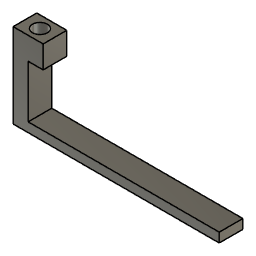
_Hook v2.cb20e67a-e10a-452d-a86b-8f95d06309be (Autodesk Fusion 360 design; units mm, degrees)
part number: 2025-05-20-10-46-20-879
part number: 2025-05-20-11-01-20-780
Autodesk Fusion 360 part; units mm, degrees
sketch "Sketch1" plane through (0, 0, 0) normal (0, 0, 1) x (1, 0, 0)
  line L0 (0, 0) -> (55, 0)
  line L1 (55, 0) -> (55, 6.3)
  line L2 (55, 6.3) -> (0, 6.3)
  line L3 (0, 6.3) -> (0, 0)
  dimension "d1" = 55
  dimension "d2" = 6.3
  constraint horizontal L0
  constraint vertical L1
  constraint horizontal L2
  constraint vertical L3
  constraint coincident L0.start L3.end
  measures "d1" distance of L0.start L0.end
  measures "d2" distance of L0.start L2.end
extrude "Extrude1" add sketch "Sketch1" along normal blind 2.5 makes body 1
sketch "Sketch2" plane through (0, 0, 2.5) normal (0, 0, 1) x (-1, 0, 0)
  line L0 (0, -6.3) -> (0, 0)
  line L1 (0, 0) -> (-55, 0)
  line L2 (-55, 0) -> (-55, -6.3)
  line L3 (-55, -6.3) -> (0, -6.3)
  line L4 (0, 0) -> (-4, 0)
  line L5 (-4, 0) -> (-4, -6.3)
  line L6 (-4, -6.3) -> (0, -6.3)
  line L7 (0, -6.3) -> (0, 0)
  dimension "d5" = 4
  constraint horizontal L4
  constraint vertical L5
  constraint horizontal L6
  constraint vertical L7
  constraint coincident L0.end L1.start
  measures "d5" distance of L0.end L4.end
extrude "Extrude2" add sketch "Sketch2" along normal blind 14 contours L0 L1 L3 L4 L5 L6 L7 bodies 1
sketch "Sketch3" plane through (0, 0, 16.5) normal (0, 0, 1) x (-1, 0, 0)
  line L0 (0, -6.3) -> (0, 0)
  line L1 (0, 0) -> (-4, 0)
  line L2 (-4, 0) -> (-4, -6.3)
  line L3 (-4, -6.3) -> (0, -6.3)
  line L4 (0, 0) -> (-8, 0)
  line L5 (-8, 0) -> (-8, -6.3)
  line L6 (-8, -6.3) -> (0, -6.3)
  line L7 (0, -6.3) -> (0, 0)
  dimension "d8" = 8
  dimension "d9" = 6.3
  constraint horizontal L4
  constraint vertical L5
  constraint horizontal L6
  constraint vertical L7
  constraint coincident L0.end L1.start
  measures "d8" distance of L0.end L4.end
  measures "d9" distance of L0.end L0.start
extrude "Extrude3" add sketch "Sketch3" along normal blind 6 bodies 1
hole "Hole1" at (4, 3.15, 22.5) direction (0, 0, -1) diameter 4 depth 4 tip angle 180 bodies 1
copy_body "Body->Comp1" bodies 1 removing the originals makes body 2 in component "Hook v2 (1)"
component "Hook v2 (1)" placed x (1, 0, 0) y (0, 1, 0) z (0, 0, 1) at (0, 0, 0)
